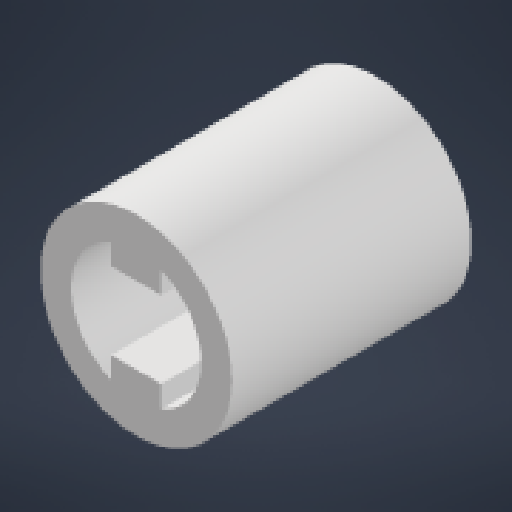
# Autodesk Inventor part: Axel_connector
Saved by Autodesk Inventor 2026 (Build 300175050, 175E)
## iProperties
Created: 2026-06-21
Part Number: Axel_connector
Material: Generic
Document SubType Name: Modeling
Designer: sniel
Density: 1 g/cm^3
Appearance: Default
Author: sniel
Autodesk Inventor part; units mm, degrees
ref_plane "YZ Plane" through (0, 0, 0) normal (1, 0, 0) x (0, 1, 0)
ref_plane "XZ Plane" through (0, 0, 0) normal (0, 1, 0) x (-1, 0, 0)
ref_plane "XY Plane" through (0, 0, 0) normal (0, 0, 1) x (1, 0, 0)
sketch "Sketch1" plane through (0, 0, 0) normal (0, 0, 1) x (1, 0, 0)
  line L0 (-3.9756, 0) -> (3.9756, 0)
  arc A0 (3.9756, 0) -> (1.5654, 3.6545) centre (0, 0) ccw
  line L1 (1.5654, 3.6545) -> (1.5654, 2.4102)
  line L2 (1.5654, 2.4102) -> (-1.5654, 2.4102)
  line L3 (-1.5654, 2.4102) -> (-1.5654, 3.6545)
  arc A1 (-1.5654, 3.6545) -> (-3.9756, 0) centre (0, 0) ccw
  circle A2 centre (0, 0) radius 4.075
  circle A3 centre (0, 0) radius 6
  line L4 (-1.5654, 3.6545) -> (-1.5654, 3.7623)
  line L5 (1.5654, 3.6545) -> (1.5654, 3.7623)
  line L6 (-4.075, 0) -> (4.2123, 0)
  line L7 (1.5654, -3.6545) -> (1.5654, -2.4102)
  line L8 (1.5654, -2.4102) -> (-1.5654, -2.4102)
  line L9 (-1.5654, -2.4102) -> (-1.5654, -3.6545)
  line L10 (-1.5654, -3.6545) -> (-1.5654, -3.7623)
  line L11 (1.5654, -3.6545) -> (1.5654, -3.7623)
  point P0 (0, 0)
  dimension "d0" = 8.15
  dimension "d1" = 12
  constraints: 24 end point, 7 point on circle, 6 symmetric about line, 4 centre point, 2 coincident, 2 vertical, 1 point on line
  measures "d0" diameter of A2
  measures "d1" diameter of A3
extrude "Extrusion1" add sketch "Sketch1" along normal blind 15 contours L4 A2 L5 L1 L2 L3 | L10 L9 L8 L7 L11 A2 | A3
body "Solid1"
